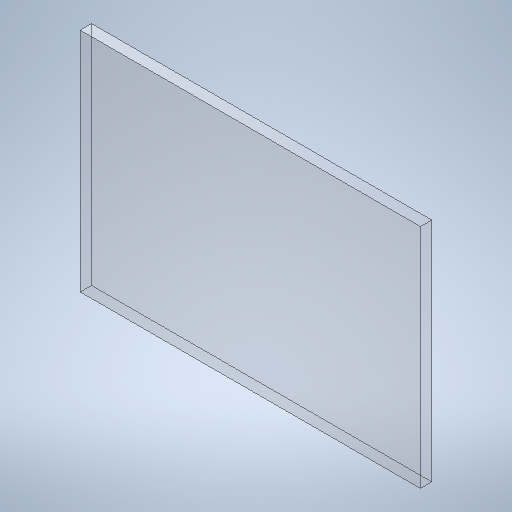
# Autodesk Inventor part: Tampo_vidro
Saved by Autodesk Inventor 2025.2 (Build 292293000, 293)
## iProperties
Created: 2025-04-07
Part Number: Tampo_vidro
Material: Vidro
Document SubType Name: Modeling
Designer: Formação
Density: 2.18 g/cm^3
Appearance: Bolhas de água
Author: Formação
Autodesk Inventor part; units mm, degrees
ref_plane "YZ Plane" through (0, 0, 0) normal (1, 0, 0) x (0, 1, 0)
ref_plane "XZ Plane" through (0, 0, 0) normal (0, 1, 0) x (-1, 0, 0)
ref_plane "XY Plane" through (0, 0, 0) normal (0, 0, 1) x (1, 0, 0)
sketch "Esboço1" plane through (0, 0, 0) normal (0, 0, 1) x (1, 0, 0)
  line L0 (-2250, 1500) -> (2250, 1500)
  line L1 (2250, 1500) -> (2250, -1500)
  line L2 (2250, -1500) -> (-2250, -1500)
  line L3 (-2250, -1500) -> (-2250, 1500)
  line L4 (-2250, 1500) -> (2250, -1500) construction
  line L5 (2250, 1500) -> (-2250, -1500) construction
  point P0 (0, 0)
  point P1 (0, 0)
  dimension "d0" = 4500
  dimension "d1" = 3000
  constraints: 12 end point, 2 coincident, 2 midpoint, 2 parallel, 1 horizontal, 1 perpendicular
  measures "d0" distance between parallel lines of L1 L3
  measures "d1" distance between parallel lines of L2 L0
extrude "Extrusão1" add sketch "Esboço1" along normal mid plane 150
